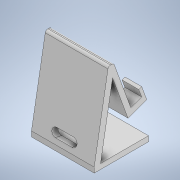
# Autodesk Inventor part: Phone Stand V3 Rev A
Saved by Autodesk Inventor 2021 (Build 250183000, 183)
## iProperties
Created: 2020-10-03
Part Number: Phone Stand V3 Rev A
Material: Generic
Document SubType Name: Modeling
Designer: cmzgt
Density: 1 g/cm^3
Appearance: Default
Author: cmzgt
Autodesk Inventor part; units mm, degrees
ref_plane "YZ Plane" through (0, 0, 0) normal (1, 0, 0) x (0, 1, 0)
ref_plane "XZ Plane" through (0, 0, 0) normal (0, 1, 0) x (-1, 0, 0)
ref_plane "XY Plane" through (0, 0, 0) normal (0, 0, 1) x (1, 0, 0)
sketch "Sketch1" plane through (0, 0, 0) normal (0, 1, 0) x (-1, 0, 0)
  line L0 (-38.1, -33.02) -> (38.1, -33.02)
  line L1 (38.1, -33.02) -> (38.1, 33.02)
  line L2 (38.1, 33.02) -> (-38.1, 33.02)
  line L3 (-38.1, 33.02) -> (-38.1, -33.02)
  line L4 (-38.1, -33.02) -> (38.1, 33.02) construction
  line L5 (38.1, -33.02) -> (-38.1, 33.02) construction
  point P0 (0, 0)
  dimension "d0" = 76.2
  dimension "d1" = 66.04
  constraints: 12 end point, 2 midpoint, 2 parallel, 1 horizontal, 1 perpendicular
  measures "d0" distance of L2.end L1.end
  measures "d1" distance of L1.end L0.end
extrude "Extrusion1" add sketch "Sketch1" along normal blind 6.35
sketch "Sketch3" plane through (38.1, 0, 33.02) normal (1, 0, 0) x (0, 0, -1)
  line L0 (66.04, 6.35) -> (0, 6.35) projected
  line L1 (0, 6.35) -> (6.35, 6.35) construction
  line L2 (0, 6.35) -> (17.2016, 103.9051)
  line L3 (17.2016, 103.9051) -> (23.6495, 103.9051)
  line L4 (23.6495, 103.9051) -> (47.1053, 39.4609)
  line L5 (47.1053, 39.4609) -> (41.1382, 37.2891)
  line L6 (41.1382, 37.2891) -> (22.3129, 89.0112)
  line L7 (22.3129, 89.0112) -> (7.7376, 6.35)
  point P0 (33.02, 0)
  dimension "d13" = 99.06
  dimension "d14" = 80
  dimension "d20" = 68.58
  dimension "d21" = 70
  dimension "d22" = 6.35
  constraints: 14 end point, 2 parallel, 2 point on line, 1 horizontal, 1 perpendicular
  measures "d13" distance of L0.end L2.end
  measures "d14" angle of L0 L2
  measures "d20" distance of L3.end L4.end
  measures "d21" angle of L0 L4
  measures "d22" distance of L4.end L5.end
extrude "Extrusion2" add sketch "Sketch3" against normal up to surface (76.2 mm away)
fillet "Fillet1" radius 3.175 2 edges at (0, 103.9051, 15.8184) (0, 103.9051, 9.3705)
sketch "Sketch6" plane through (38.1, 39.4609, -14.0853) normal (0, 0.3420201, -0.9396926) x (-1, 0, 0)
  line L0 (0, 0) -> (0, 66.3568) projected
  line L1 (0, 0) -> (20.32, 0)
  line L2 (20.32, 0) -> (20.32, 7.62)
  line L3 (20.32, 7.62) -> (0, 7.62)
  line L4 (0, 7.62) -> (0, 0)
  line L5 (0, 66.3568) -> (76.2, 66.3568) projected
  line L6 (38.1, 66.3568) -> (38.1, 0)
  line L7 (0, 0) -> (76.2, 0) projected
  line L8 (76.2, 0) -> (55.88, 0)
  line L9 (55.88, 0) -> (55.88, 7.62)
  line L10 (55.88, 7.62) -> (76.2, 7.62)
  line L11 (76.2, 0) -> (76.2, 66.3568) projected
  line L12 (76.2, 7.62) -> (76.2, 0)
  point P0 (38.1, -32.2637)
  point P1 (55.88, 0)
  point P2 (0, 7.62)
  dimension "d24" = 20.32
  dimension "d25" = 7.62
  constraints: 18 end point, 3 symmetric about line, 2 midpoint, 2 parallel, 1 collinear, 1 horizontal, 1 perpendicular
  measures "d24" distance of L3.end L2.end
  measures "d25" distance of L1.end L2.end
extrude "Extrusion3" add sketch "Sketch6" along normal blind 17.78 contours L0 L3 L2 L1 | L9 L10 L11 L7
sketch "Sketch7" plane through (17.78, 46.6214, -11.4791) normal (0, 0.9396926, 0.3420201) x (1, 0, 0)
  line L0 (0, 17.78) -> (20.32, 17.78) projected
  line L1 (20.32, 17.78) -> (0, 17.78)
  line L2 (0, 17.78) -> (0, 13.97)
  line L3 (0, 13.97) -> (20.32, 13.97)
  line L4 (20.32, 13.97) -> (20.32, 17.78)
  line L5 (20.32, -3.5556) -> (-55.88, -3.5556) projected
  line L6 (-17.78, -3.5556) -> (-17.78, 27.2379)
  line L7 (-35.56, 17.78) -> (-55.88, 17.78)
  line L8 (-35.56, 17.78) -> (-35.56, 13.97)
  line L9 (-35.56, 13.97) -> (-55.88, 13.97)
  line L10 (-55.88, 13.97) -> (-55.88, 17.78)
  point P0 (-17.78, -26.7323)
  dimension "d28" = 3.81
  constraints: 18 end point, 5 symmetric about line, 2 parallel, 1 horizontal, 1 midpoint, 1 perpendicular, 1 vertical
  measures "d28" distance of L2.end L1.end
extrude "Extrusion4" add sketch "Sketch7" along normal blind 10.16
sketch "Sketch8" plane through (-38.1, 6.35, 33.02) normal (0, 0.1736482, 0.9848078) x (1, 0, 0)
  line L0 (48.26, 11.4677) -> (27.94, 11.4677) construction
  line L1 (76.2, 11.4677) -> (0, 11.4677) projected
  line L2 (48.26, 16.5477) -> (27.94, 16.5477)
  line L3 (27.94, 6.3877) -> (48.26, 6.3877)
  arc A0 (48.26, 6.3877) -> (48.26, 16.5477) centre (48.26, 11.4677) ccw
  arc A1 (27.94, 16.5477) -> (27.94, 6.3877) centre (27.94, 11.4677) ccw
  point P0 (38.1, -0.5197)
  point P1 (38.1, 11.4677)
  dimension "d31" = 10.16
  dimension "d32" = 10.16
  constraints: 8 end point, 4 point on circle, 4 tangent, 2 centre point, 2 midpoint, 1 parallel, 1 point on line
  measures "d31" distance of point (38.1, 11.468) L0.end
  measures "d32" diameter of A1
extrude "Extrusion5" cut sketch "Sketch8" against normal blind 10.16
body "Solid1"
